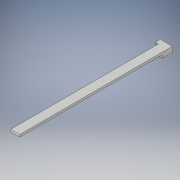
# Autodesk Inventor part: rails
Saved by Autodesk Inventor 2017 (Build 210142000, 142)
## iProperties
Created: 2018-11-15
Part Number: rails
Material: Generic
Document SubType Name: Modeling
Designer: Antoine Blaud
Density: 1 g/cm^3
Appearance: Default
Author: Antoine Blaud
Autodesk Inventor part; units mm, degrees
ref_plane "YZ Plane" through (0, 0, 0) normal (1, 0, 0) x (0, 1, 0)
ref_plane "XZ Plane" through (0, 0, 0) normal (0, 1, 0) x (-1, 0, 0)
ref_plane "XY Plane" through (0, 0, 0) normal (0, 0, 1) x (1, 0, 0)
sketch "Sketch1" plane through (0, 0, 0) normal (1, 0, 0) x (0, 1, 0)
  line L0 (0, 0) -> (3.81, 0)
  line L1 (3.81, 0) -> (3.81, -254)
  line L2 (3.81, -254) -> (0, -254)
  line L3 (0, -254) -> (0, 0)
  dimension "d0" = 254
  dimension "d1" = 3.81
  constraints: 8 end point, 2 parallel, 1 horizontal, 1 perpendicular
  measures "d0" distance of L0.end L1.end
  measures "d1" distance of L0.start L0.end
extrude "Extrusion1" add sketch "Sketch1" along normal blind 15
sketch "Sketch2" plane through (0, 0, -254) normal (0, -1, 0) x (1, 0, 0)
  line L0 (15, 254) -> (15, 0) projected
  line L1 (0, 0) -> (0, 254) projected
  line L2 (15, 0) -> (0, 0)
  line L3 (0, 0) -> (0, 17.0864)
  line L4 (0, 17.0864) -> (15, 17.0864)
  line L5 (15, 17.0864) -> (15, 0)
  dimension "d4" = 17.0864
  constraints: 8 end point, 2 parallel, 1 horizontal, 1 perpendicular, 1 point on line
  measures "d4" distance between parallel lines of L2 L4
extrude "Extrusion2" add sketch "Sketch2" along normal blind 5.08
sketch "Sketch3" plane through (0, 0, 0) normal (-1, 0, 0) x (0, 0, 1)
  line L0 (-254, 3.81) -> (-254, -5.08) projected
  line L1 (0, 3.81) -> (-254, 3.81) projected
  line L2 (-254, -5.08) -> (-245.8991, -5.08)
  line L3 (-245.8991, -5.08) -> (-245.8991, 3.81)
  line L4 (-245.8991, 3.81) -> (-254, 3.81)
  line L5 (-254, 3.81) -> (-254, -5.08)
  point P0 (0, 0)
  dimension "d7" = 8.1008
  constraints: 8 end point, 2 parallel, 1 horizontal, 1 perpendicular, 1 point on line
  measures "d7" distance between parallel lines of L0 L3
extrude "Extrusion3" add sketch "Sketch3" along normal blind 5.08
body "Solid1"
